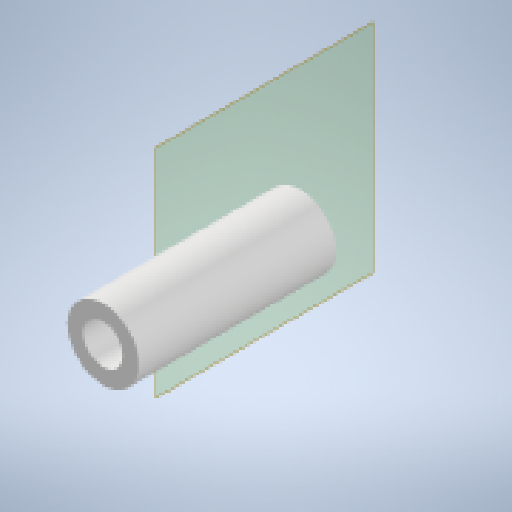
# Autodesk Inventor part: MotorMountSpacerConnector
Saved by Autodesk Inventor 2024 (Build 280153020, 153B)
## iProperties
Created: 2024-04-18
Part Number: MotorMountSpacerConnector
Material: Generic
Document SubType Name: Modeling
Designer: lvrectanus0
Density: 1 g/cm^3
Appearance: Default
Author: lvrectanus0
Autodesk Inventor part; units mm, degrees
ref_plane "YZ Plane" through (0, 0, 0) normal (1, 0, 0) x (0, 1, 0)
ref_plane "XZ Plane" through (0, 0, 0) normal (0, 1, 0) x (-1, 0, 0)
ref_plane "XY Plane" through (0, 0, 0) normal (0, 0, 1) x (1, 0, 0)
sketch "Sketch1" plane through (0, 0, 0) normal (0, 0, 1) x (1, 0, 0)
  line L0 (3.526, -23.5864) -> (6.6455, -8.4436) projected
  arc A0 (16.2171, 4.4559) -> (6.6455, -8.4436) centre (25.3037, -12.2874) ccw projected
  arc A1 (16.2171, 4.4559) -> (17.3448, 5.4138) centre (14.5, 7.62) ccw projected
  line L1 (17.3448, 5.4138) -> (28.7885, 20.1696) projected
  arc A2 (28.7885, 20.1696) -> (25.2625, 26.2768) centre (26.3965, 22.86) ccw projected
  line L2 (25.2625, 26.2768) -> (9.9483, 21.1944) projected
  arc A3 (1.5903, 20.3712) -> (9.9483, 21.1944) centre (3.9479, 39.2748) ccw projected
  arc A4 (1.5903, 20.3712) -> (-1.5903, 20.3712) centre (0, 7.62) ccw projected
  arc A5 (-9.9483, 21.1944) -> (-1.5903, 20.3712) centre (-3.9479, 39.2748) ccw projected
  line L3 (-9.9483, 21.1944) -> (-25.2625, 26.2768) projected
  arc A6 (-25.2625, 26.2768) -> (-28.7885, 20.1696) centre (-26.3965, 22.86) ccw projected
  line L4 (-28.7885, 20.1696) -> (-17.3448, 5.4138) projected
  arc A7 (-17.3448, 5.4138) -> (-16.2171, 4.4559) centre (-14.5, 7.62) ccw projected
  arc A8 (-6.6455, -8.4436) -> (-16.2171, 4.4559) centre (-25.3037, -12.2874) ccw projected
  line L5 (-6.6455, -8.4436) -> (-3.526, -23.5864) projected
  arc A9 (-3.526, -23.5864) -> (3.526, -23.5864) centre (0, -22.86) ccw projected
  circle A10 centre (0, -22.86) radius 2 projected
  circle A11 centre (0, 7.62) radius 9.75 projected
  circle A12 centre (14.5, 7.62) radius 2 projected
  circle A13 centre (-14.5, 7.62) radius 2 projected
  circle A14 centre (-26.3965, 22.86) radius 2 projected
  circle A15 centre (26.3965, 22.86) radius 2 projected
  circle A16 centre (0, -22.86) radius 3.6
  circle A17 centre (0, -22.86) radius 2
  point P0 (0, 0)
  point P1 (-3.6, -22.86)
  constraints: 2 coincident, 1 centre point, 1 concentric, 1 horizontal alignment, 4 other
extrude "Extrusion1" add sketch "Sketch1" along normal blind 20 contours A9 A16
ref_plane "Work Plane1" through (-3.6, -22.86, 0) normal (-1, 0, 0) x (0, -1, 0)
sketch "Sketch2" plane through (-3.6, -22.86, 0) normal (-1, 0, 0) x (0, -1, 0)
  line L0 (3.6, 20) -> (-3.6, 20) projected
  line L1 (3.6, 0) -> (-3.6, 0) projected
  line L2 (-3.6, 0) -> (-3.6, 20) construction
  circle A0 centre (-7.2, 10) radius 3.6
  circle A1 centre (-7.2, 10) radius 4.4
  point P0 (-22.86, 0)
  point P1 (-3.6, 10)
  dimension "d2" = 7.2
  dimension "d5" = 0.8
  constraints: 2 centre point, 2 end point, 1 horizontal alignment, 1 midpoint, 1 tangent, 1 vertical
  measures "d2" diameter of A0
  measures "d5" radial gap between concentric circles of A0 A1
extrude "Extrusion2" add sketch "Sketch2" against normal blind 7.2 contours A0 | A1
fillet "Fillet1" radius 1 2 edges at (0.0008, -19.26, 12.5298) (0.0008, -19.26, 7.4702)
sketch "Sketch3" plane through (-3.6, -22.86, 0) normal (-1, 0, 0) x (0, 0, 1)
  arc A0 (12.622, 3.6666) -> (7.378, 3.6666) centre (10, 7.2) ccw projected
  point P0 (0, 22.86)
  constraints: 1 coincident, 1 horizontal alignment
hole "Hole1" at (-3.6, -15.66, 10) direction (1, 0, 0) diameter 4 depth 6
body "Solid1"
